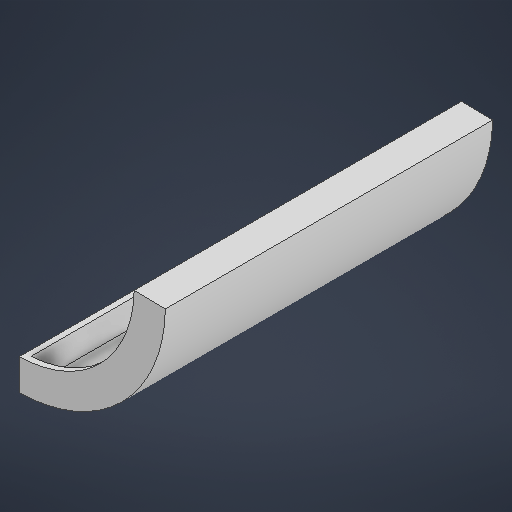
# Autodesk Inventor part: shim_former
Saved by Autodesk Inventor 2026.1 (Build 301233020, 233B)
## iProperties
Created: 2025-11-19
Part Number: shim_former
Material: Generic
Document SubType Name: Modeling
Designer: Carla Fernandez
Density: 1 g/cm^3
Appearance: Default
Author: Carla Fernandez
Autodesk Inventor part; units mm, degrees
ref_plane "Work Plane1" through (0, 0, 87) normal (0, 0, 1) x (1, 0, 0)
ref_plane "YZ Plane" through (0, 0, 0) normal (1, 0, 0) x (0, 1, 0)
ref_plane "XZ Plane" through (0, 0, 0) normal (0, 1, 0) x (-1, 0, 0)
sketch "Sketch4" plane through (0, 0, 0) normal (0, 0, 1) x (1, 0, 0)
  arc A0 (1.3264, -75.9884) -> (75.9884, -1.3264) centre (0, 0) ccw
  arc A1 (1.0471, -59.9909) -> (59.9909, -1.0471) centre (0, 0) ccw
  line L0 (0, -92.1462) -> (0, 0) construction
  line L1 (0, 0) -> (129.1278, 0) construction
  line L2 (0, 0) -> (106.82, -1.8646) construction
  line L3 (0, 0) -> (1.3871, -79.4693) construction
  line L4 (1.0471, -59.9909) -> (1.3264, -75.9884)
  line L5 (59.9909, -1.0471) -> (75.9884, -1.3264)
  dimension "d33" = 152
  dimension "d34" = 120
  dimension "d35" = 1
  dimension "d36" = 1
  constraints: 12 end point, 4 point on circle, 4 point on line, 2 centre point, 2 coincident, 1 perpendicular, 1 vertical
  measures "d33" diameter of A0
  measures "d34" diameter of A1
  measures "d35" angle of L1 L2
  measures "d36" angle of L3 L0
extrude "Extrusion3" add sketch "Sketch4" along normal mid plane 168
shell "Shell2" thickness 3 removed faces 1 at (4.4562, -59.8343, 28)
sketch "Sketch1" plane through (0, 0, 0) normal (0, 0, 1) x (1, 0, 0)
  circle A0 centre (0, 0) radius 77.5
  circle A1 centre (0, 0) radius 76.5
  dimension "d0" = 155
  dimension "d1" = 153
  constraints: 2 centre point, 2 coincident
  measures "d0" diameter of A0
  measures "d1" diameter of A1
sketch "Sketch2" plane through (0, 0, 87) normal (0, 0, 1) x (1, 0, 0)
  line L0 (0, 0) -> (0, -91.1898) construction
  line L1 (0, 0) -> (8.9718, -102.5486) construction
  arc A0 (7.9909, -74.1258) -> (5.0023, -74.3873) centre (6.2752, -71.726) ccw
  line L2 (5.0023, -74.3873) -> (5.1718, -76.325)
  line L3 (7.9909, -74.1258) -> (8.1604, -76.0635)
  circle A1 centre (0, 0) radius 76.5 projected
  arc A2 (5.1718, -76.325) -> (8.1604, -76.0635) centre (0, 0) ccw
  line L4 (7.9909, -74.1258) -> (0, 0) construction
  line L5 (0, 0) -> (5.0023, -74.3873) construction
  line L6 (0, 0) -> (93.5228, -13.1438) construction
  line L7 (0, 0) -> (97.964, 0) construction
  circle A3 centre (0, 0) radius 76.5
  line L8 (68, 0) -> (76.5, 0)
  line L9 (67.3382, -9.4638) -> (75.7555, -10.6467)
  arc A4 (67.3382, -9.4638) -> (68, 0) centre (0, 0) ccw
  point P0 (75.7555, -10.6467)
  dimension "d5" = 5
  dimension "d6" = 5.9
  dimension "d7" = 72
  dimension "d8" = 3
  dimension "d12" = 8
  dimension "d32" = 68
  constraints: 20 end point, 10 point on circle, 4 centre point, 4 parallel, 3 coincident, 3 point on line, 2 concentric, 1 collinear, 1 horizontal, 1 vertical
  measures "d5" angle of L1 L0
  measures "d6" diameter of A0
  measures "d7" distance of A0.centre L0.start
  measures "d8" distance between parallel lines of L3 L2
  measures "d12" angle of L6 L7
  measures "d32" radius of A4
sketch "Sketch3" plane through (75.7555, -10.6467, 84) normal (-0.1392, -0.9903, 0) x (0.9903, -0.1392, 0)
  line L0 (-8.1618, 1) -> (0, 1)
  line L1 (0, 1) -> (0, 5)
  line L2 (0, 5) -> (-8.1618, 5)
  line L3 (-8.1618, 5) -> (-8.1618, 1)
  line L4 (0, 6) -> (0, -174) construction
  line L5 (0, -1.3495) -> (0, 7.9011) construction
  line L6 (-9.1618, 0) -> (-0.7445, 0) construction
  line L7 (-0.7445, 6) -> (-9.1618, 6) construction
  line L8 (-9.1618, 6) -> (-9.1618, 0) construction
  line L9 (-76.5, -210.3802) -> (-76.5, 44.2814) projected
  point P0 (-76.5, -84)
  dimension "d23" = 1
  dimension "d24" = 1
  dimension "d25" = 1
  constraints: 10 end point, 2 parallel, 1 collinear, 1 horizontal, 1 perpendicular, 1 point on line, 1 vertical
  measures "d23" distance between parallel lines of L0 L6
  measures "d24" distance between parallel lines of L7 L2
  measures "d25" distance between parallel lines of L8 L3
body "Solid1"
body "Solid2"
